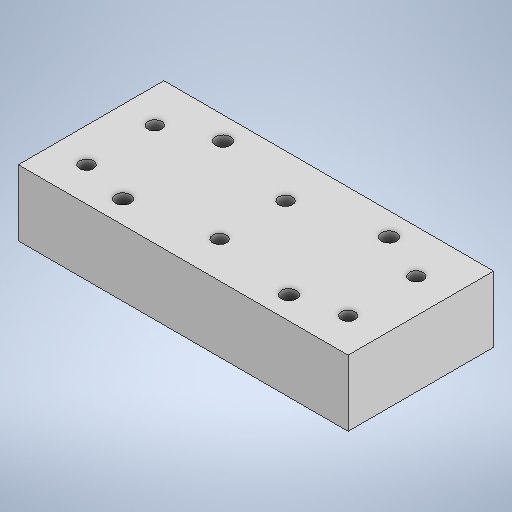
# Autodesk Inventor part: assist_wheel_bracket
Saved by Autodesk Inventor 2026.2 (Build 302298010, 298A)
## iProperties
Created: 2026-04-05
Part Number: assist_wheel_bracket
Material: Generic
Document SubType Name: Modeling
Designer: chanh
Density: 1 g/cm^3
Appearance: Default
Author: chanh
Autodesk Inventor part; units mm, degrees
ref_plane "YZ Plane" through (0, 0, 0) normal (1, 0, 0) x (0, 1, 0)
ref_plane "XZ Plane" through (0, 0, 0) normal (0, 1, 0) x (-1, 0, 0)
ref_plane "XY Plane" through (0, 0, 0) normal (0, 0, 1) x (1, 0, 0)
sketch "Sketch1" plane through (0, 0, 0) normal (0, 1, 0) x (-1, 0, 0)
  line L0 (72.5, 32) -> (-72.5, 32)
  line L1 (-72.5, 32) -> (-72.5, -32)
  line L2 (-72.5, -32) -> (72.5, -32)
  line L3 (72.5, -32) -> (72.5, 32)
  line L4 (72.5, 32) -> (-72.5, -32) construction
  line L5 (-72.5, 32) -> (72.5, -32) construction
  line L6 (0, 0) -> (0, -32) construction
  line L7 (0, 0) -> (0, 32) construction
  circle A0 centre (0, -13) radius 3.05
  circle A1 centre (0, 16) radius 3.05
  circle A2 centre (57.5, -13) radius 3.05
  circle A3 centre (57.5, 17) radius 3.05
  line L8 (57.5, -13) -> (57.5, 17) construction
  circle A4 centre (-57.5, -13) radius 3.05
  circle A5 centre (-57.5, 17) radius 3.05
  point P0 (57.5, 2)
  dimension "d0" = 145
  dimension "d1" = 64
  dimension "d2" = 6.1
  dimension "d3" = 6.1
  dimension "d4" = 15
  dimension "d5" = 30
  dimension "d18" = 2
  constraints: 18 end point, 6 centre point, 6 midpoint, 2 equal radius, 2 parallel, 2 symmetric about line, 1 horizontal, 1 horizontal alignment, 1 perpendicular, 1 point on line, 1 vertical, 1 vertical alignment, 2 other
  measures "d0" distance of L2.end L1.end
  measures "d1" distance of L1.end L0.end
  measures "d2" diameter of A0
  measures "d3" diameter of A2
  measures "d4" distance between parallel lines of L3 L8
  measures "d5" distance of L8.start L8.end
  measures "d18" vertical distance of point (57.5, 2) L6.start
extrude "Extrusion1" add sketch "Sketch1" along normal blind 29
sketch "Sketch2" plane through (0, 0, 0) normal (0, -1, 0) x (1, 0, 0)
  arc A0 (-35.5, 17.5) -> (-35.5, 26.5) centre (-35.5, 22) ccw projected
  line L0 (-37.5, 17.5) -> (-35.5, 17.5) projected
  arc A1 (-37.5, 26.5) -> (-37.5, 17.5) centre (-37.5, 22) ccw projected
  line L1 (-35.5, 26.5) -> (-37.5, 26.5) projected
  line L2 (-35.5, -17.5) -> (-37.5, -17.5) projected
  arc A2 (-35.5, -26.5) -> (-35.5, -17.5) centre (-35.5, -22) ccw projected
  line L3 (-37.5, -26.5) -> (-35.5, -26.5) projected
  arc A3 (-37.5, -17.5) -> (-37.5, -26.5) centre (-37.5, -22) ccw projected
  line L4 (35.5, -26.5) -> (37.5, -26.5) projected
  arc A4 (35.5, -17.5) -> (35.5, -26.5) centre (35.5, -22) ccw projected
  line L5 (37.5, -17.5) -> (35.5, -17.5) projected
  arc A5 (37.5, -26.5) -> (37.5, -17.5) centre (37.5, -22) ccw projected
  line L6 (37.5, 26.5) -> (35.5, 26.5) projected
  arc A6 (37.5, 17.5) -> (37.5, 26.5) centre (37.5, 22) ccw projected
  line L7 (35.5, 17.5) -> (37.5, 17.5) projected
  arc A7 (35.5, 26.5) -> (35.5, 17.5) centre (35.5, 22) ccw projected
  circle A8 centre (36.5, 0) radius 4.5 projected
  circle A9 centre (-36.5, 0) radius 4.5 projected
  line L8 (47, -32) -> (-47, -32) projected
  line L9 (47, 32) -> (47, -32) projected
  line L10 (-47, 32) -> (47, 32) projected
  line L11 (-47, -32) -> (-47, 32) projected
  circle A10 centre (0, 0) radius 20 projected
  line L12 (-37.5, -22) -> (-35.5, -22)
  line L13 (35.5, -22) -> (37.5, -22)
  line L14 (35.5, 22) -> (37.5, 22)
  line L15 (-37.5, 22) -> (-35.5, 22)
  point P0 (0, 0)
  point P1 (-36.5, -22)
  point P2 (-36.5, 22)
  point P3 (36.5, 22)
  point P4 (36.5, -22)
  constraints: 8 end point, 4 horizontal, 4 midpoint
hole "Hole1" at (-36.5, 0, -22) at (-36.5, 0, 22) at (36.5, 0, 22) at (36.5, 0, -22) direction (0, 1, 0) diameter 6.647 end through all thread size "M8x1.25" class "6H" standard "ISO Metric profile"
sketch "Sketch4" plane through (0, 0, 0) normal (0, -1, 0) x (1, 0, 0)
  circle A0 centre (-57.5, 17) radius 3.05 projected
  circle A1 centre (-57.5, -13) radius 3.05 projected
  circle A2 centre (0, -13) radius 3.05 projected
  circle A3 centre (0, 16) radius 3.05 projected
  circle A4 centre (57.5, 17) radius 3.05 projected
  circle A5 centre (57.5, -13) radius 3.05 projected
  circle A6 centre (-57.5, 17) radius 6
  circle A7 centre (-57.5, -13) radius 6
  circle A8 centre (0, 16) radius 6
  circle A9 centre (0, -13) radius 6
  circle A10 centre (57.5, 17) radius 6
  circle A11 centre (57.5, -13) radius 6
  point P0 (0, 0)
  dimension "d15" = 12
  constraints: 6 centre point, 6 coincident, 5 equal radius
  measures "d15" diameter of A6
extrude "Extrusion2" cut sketch "Sketch4" against normal blind 6 contours A0 | A1 | A2 | A3 | A4 | A5 | A6 | A7 | A8 | A9 | A10 | A11
body "Solid1"
